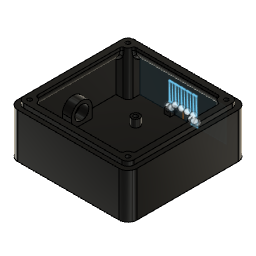
CO2 Melder RG Projekt 2 überarbeitung v13 (Autodesk Fusion 360 design; units mm, degrees)
Autodesk Fusion 360 part; units mm, degrees
sketch "Skizze1" plane through (0, 0, 0) normal (0, 0, 1) x (1, 0, 0)
  line L0 (0, 0) -> (80, 0)
  line L1 (80, 0) -> (80, 80)
  line L2 (80, 80) -> (0, 80)
  line L3 (0, 80) -> (0, 0)
  dimension "d1" = 80
  dimension "d2" = 80
  constraint horizontal L0
  constraint vertical L1
  constraint horizontal L2
  constraint vertical L3
  constraint coincident L0.start L3.end
  measures "d1" distance of L0.start L0.end
  measures "d2" distance of L0.start L2.end
extrude "Extrusion1" add sketch "Skizze1" along normal blind 30
shell "Schale1" thickness 3 removed faces 1 at (26.6667, 53.3333, 30)
sketch "Skizze2" plane through (0, 0, 3) normal (0, 0, 1) x (-1, 0, 0)
  line L0 (-3, -77) -> (-3, -3)
  line L1 (-3, -3) -> (-77, -3)
  line L2 (-77, -3) -> (-77, -77)
  line L3 (-77, -77) -> (-3, -77)
  line L4 (-27.15, -58) -> (-52.85, -58) construction
  line L5 (-52.85, -58) -> (-52.85, -5.7) construction
  line L6 (-52.85, -5.7) -> (-27.15, -5.7) construction
  line L7 (-27.15, -5.7) -> (-27.15, -58) construction
  circle A0 centre (-27.15, -58) radius 1.4
  circle A1 centre (-52.85, -58) radius 1.4
  circle A2 centre (-27.15, -5.7) radius 1.4
  circle A3 centre (-52.85, -5.7) radius 1.4
  circle A4 centre (-27.15, -5.7) radius 2.75
  circle A5 centre (-27.15, -58) radius 2.75
  circle A6 centre (-52.85, -58) radius 2.75
  circle A7 centre (-52.85, -5.7) radius 2.75
  line L8 (-3, -3) -> (-77, -77) construction
  line L9 (-3, -3) -> (-5, -5) construction
  line L10 (-3, -3) -> (-18.5563, -18.5563) construction
  line L11 (-77, -77) -> (-61.4437, -61.4437) construction
  circle A8 centre (-18.5563, -18.5563) radius 5
  circle A9 centre (-61.4437, -61.4437) radius 5
  dimension "d7" = 25.7
  dimension "d8" = 52.3
  dimension "d9" = 2.8
  dimension "d10" = 2.8
  dimension "d11" = 2.8
  dimension "d12" = 2.8
  dimension "d13" = 5.5
  dimension "d14" = 5.5
  dimension "d15" = 5.5
  dimension "d16" = 5.5
  dimension "d88" = 22
  dimension "d90" = 22
  dimension "d91" = 10
  dimension "d92" = 10
  constraint horizontal L4
  constraint vertical L5
  constraint horizontal L6
  constraint vertical L7
  constraint coincident L4.start L7.end
  constraint coincident L4.end L5.start
  constraint coincident L6.end L7.start
  constraint coincident L5.end L6.start
  constraint concentric A2 A4
  constraint concentric A0 A5
  constraint concentric A1 A6
  constraint concentric A3 A7
  constraint coincident L0.end L1.start
  constraint coincident L2.end L3.start
  constraint coincident L8 L9.end
  constraint parallel L8 L10
  constraint coincident L10.end A8.centre
  constraint coincident L11.end A9.centre
  measures "d7" distance of L4.start L4.end
  measures "d8" distance of L4.start L6.end
  measures "d9" diameter of A0
  measures "d10" diameter of A1
  measures "d11" diameter of A2
  measures "d12" diameter of A3
  measures "d13" diameter of A4
  measures "d14" diameter of A5
  measures "d15" diameter of A6
  measures "d16" diameter of A7
  measures "d88" distance of L0.end L10.end
  measures "d90" distance of L2.end L11.end
  measures "d91" diameter of A8
  measures "d92" diameter of A9
extrude "Extrusion2" add sketch "Skizze2" along normal blind 5 contours L1 A4 | L1 A4 | L1 A7 | L1 A7 | A5 | A6
extrude "Extrusion11" add sketch "Skizze2" along normal blind 1 contours A8 | A9
fillet "Abrundung1" radius 6 4 edges at (0, 0, 15) (0, 80, 15) (80, 80, 15) (80, 0, 15)
fillet "Abrundung2" radius 4 4 edges at (77, 3, 16.5) (3, 3, 16.5) (3, 77, 16.5) (77, 77, 16.5)
ref_plane "Arbeitsebene1" through (0, 0, 33) normal (0, 0, 1) x (1, 0, 0)
sketch "Skizze3" plane through (40, 40, 33) normal (0, 0, 1) x (1, 0, 0)
  line L0 (-33, -37) -> (33, -37)
  line L1 (37, -33) -> (37, 33)
  line L2 (33, 37) -> (-33, 37)
  line L3 (-37, 33) -> (-37, -33)
  line L4 (-29, -33) -> (29, -33)
  line L5 (33, -29) -> (33, 29)
  line L6 (29, 33) -> (-29, 33)
  line L7 (-33, 29) -> (-33, -29)
  arc A0 (-29, 33) -> (-33, 29) centre (-29, 29) ccw
  arc A1 (-33, -29) -> (-29, -33) centre (-29, -29) ccw
  arc A2 (29, -33) -> (33, -29) centre (29, -29) ccw
  arc A3 (33, 29) -> (29, 33) centre (29, 29) ccw
  arc A4 (-37, -33) -> (-33, -37) centre (-33, -33) ccw
  arc A5 (33, -37) -> (37, -33) centre (33, -33) ccw
  arc A6 (37, 33) -> (33, 37) centre (33, 33) ccw
  arc A7 (-33, 37) -> (-37, 33) centre (-33, 33) ccw
  circle A8 centre (-33, -33) radius 1.4
  circle A9 centre (33, -33) radius 1.4
  circle A10 centre (-33, 33) radius 1.4
  circle A11 centre (33, 33) radius 1.4
  line L8 (37, 37) -> (29, 37)
  line L9 (29, 37) -> (29, 32)
  line L10 (32.3, 28.7) -> (37, 28.7)
  line L11 (37, 28.7) -> (37, 37)
  arc A12 (29, 32) -> (32.3, 28.7) centre (32.3, 32) ccw
  line L12 (-37, 37) -> (-29, 37)
  line L13 (-29, 37) -> (-29, 32.3)
  line L14 (-32.3, 29) -> (-37, 29)
  line L15 (-37, 29) -> (-37, 37)
  arc A13 (-32.3, 29) -> (-29, 32.3) centre (-32.3, 32.3) ccw
  line L16 (-32.3, -29) -> (-37, -29)
  line L17 (-37, -29) -> (-37, -37)
  line L18 (-37, -37) -> (-29, -37)
  line L19 (-29, -37) -> (-29, -32.3)
  arc A14 (-29, -32.3) -> (-32.3, -29) centre (-32.3, -32.3) ccw
  line L20 (37, -37) -> (29, -37)
  line L21 (29, -37) -> (29, -32.3)
  line L22 (32.3, -29) -> (37, -29)
  line L23 (37, -29) -> (37, -37)
  arc A15 (32.3, -29) -> (29, -32.3) centre (32.3, -32.3) ccw
  line L24 (-34, 40) -> (34, 40)
  line L25 (40, 34) -> (40, -34)
  line L26 (34, -40) -> (-34, -40)
  line L27 (-40, -34) -> (-40, 34)
  arc A16 (-34, 40) -> (-40, 34) centre (-34, 34) ccw
  arc A17 (40, 34) -> (34, 40) centre (34, 34) ccw
  arc A18 (34, -40) -> (40, -34) centre (34, -34) ccw
  arc A19 (-40, -34) -> (-34, -40) centre (-34, -34) ccw
  point P0 (33, -33)
  point P1 (-33, 33)
  point P2 (-33, -33)
  dimension "d22" = 66
  dimension "d23" = 66
  dimension "d26" = 4
  dimension "d29" = 4
  dimension "d36" = 2.8
  dimension "d37" = 2.8
  dimension "d38" = 2.8
  dimension "d39" = 2.8
  dimension "d48" = 3.3
  dimension "d49" = 3.3
  dimension "d50" = 3.3
  dimension "d51" = 3.3
  dimension "d97" = 6
  constraint horizontal L0
  constraint vertical L1
  constraint horizontal L2
  constraint vertical L3
  constraint horizontal L4
  constraint vertical L5
  constraint horizontal L6
  constraint vertical L7
  constraint coincident P1 L6
  constraint coincident P1 L7
  constraint tangent L6 A0
  constraint tangent L7 A0
  constraint coincident L4 P2
  constraint coincident L7 P2
  constraint tangent L4 A1
  constraint tangent L7 A1
  constraint equal A0 A1
  constraint coincident P0 L4
  constraint coincident P0 L5
  constraint tangent L4 A2
  constraint tangent L5 A2
  constraint equal A0 A2
  constraint tangent L5 A3
  constraint tangent L6 A3
  constraint equal A0 A3
  constraint tangent L0 A4
  constraint tangent L3 A4
  constraint tangent L0 A5
  constraint tangent L1 A5
  constraint equal A4 A5
  constraint tangent L1 A6
  constraint tangent L2 A6
  constraint equal A4 A6
  constraint tangent L2 A7
  constraint tangent L3 A7
  constraint equal A4 A7
  constraint coincident P2 A4.centre
  constraint concentric A5 A9
  constraint coincident P1 A7.centre
  constraint concentric A6 A11
  constraint horizontal L8
  constraint vertical L9
  constraint horizontal L10
  constraint vertical L11
  constraint tangent L9 A12
  constraint tangent L10 A12
  constraint horizontal L12
  constraint vertical L13
  constraint horizontal L14
  constraint vertical L15
  constraint tangent L13 A13
  constraint tangent L14 A13
  constraint horizontal L16
  constraint vertical L17
  constraint horizontal L18
  constraint vertical L19
  constraint tangent L16 A14
  constraint tangent L19 A14
  constraint horizontal L20
  constraint vertical L21
  constraint horizontal L22
  constraint vertical L23
  constraint tangent L21 A15
  constraint tangent L22 A15
  constraint horizontal L24
  constraint vertical L25
  constraint horizontal L26
  constraint vertical L27
  constraint tangent L24 A16
  constraint tangent L27 A16
  constraint tangent L24 A17
  constraint tangent L25 A17
  constraint equal A16 A17
  constraint tangent L25 A18
  constraint tangent L26 A18
  constraint equal A16 A18
  constraint tangent L26 A19
  constraint tangent L27 A19
  constraint equal A16 A19
  measures "d22" distance of P0 P2
  measures "d23" distance of P1 A4.centre
  measures "d26" radius of A0
  measures "d29" radius of A4
  measures "d36" diameter of A8
  measures "d37" diameter of A9
  measures "d38" diameter of A10
  measures "d39" diameter of A11
  measures "d48" radius of A12
  measures "d49" radius of A13
  measures "d50" radius of A14
  measures "d51" radius of A15
  measures "d97" radius of A16
extrude "Extrusion3" add sketch "Skizze3" against normal blind 8 contours L0 L3 A1 A4 L16 L17 L18 L19 | L0 L4 L19 L21 | L0 L1 A2 A5 L20 L21 L22 L23 | L3 L7 L14 L16 | L2 L3 A0 A7 L12 L13 L14 L15 | L1 L5 L10 L22 | L1 L2 L5 A3 A6 L8 L9 L10 L11 | L2 L6 L9 L13 | A8 | A9 | A10 | A11
extrude "Extrusion4" add sketch "Skizze3" against normal blind 30 contours L0 L3 A1 A4 L16 L17 L18 L19 | L0 L1 A2 A5 L20 L21 L22 L23 | A1 L16 L19 A14 | A2 L21 L22 A15 | L2 L3 A0 A7 L12 L13 L14 L15 | A0 L13 L14 A13 | L5 A3 L9 L10 A12 | L1 L2 L5 A3 A6 L8 L9 L10 L11
extrude "Extrusion5" cut sketch "Skizze3" against normal blind 10 contours A8 | A9 | A10 | A11
fillet "Abrundung3" radius 6.5 4 edges at (73, 39.85, 25) (40, 73, 25) (40, 7, 25) (7, 40, 25)
fillet "Abrundung4" radius 1.5 16 edges at (11, 73, 32) (11, 74.0917, 27.3944) (7, 69, 32) (5.9083, 69, 27.3944) (73, 11, 32) (74.0917, 11, 27.3944) (69, 7, 32) (69, 5.9083, 27.3944) (11, 7, 32) (11, 5.9083, 27.3944) (7, 11, 32) (5.9083, 11, 27.3944) (69, 73, 32) (69, 74.0917, 27.3944) (73, 68.7, 32) (74.0917, 68.7, 27.3944)
sketch "Skizze4" plane through (3, 0, 0) normal (1, 0, 0) x (0, 1, 0)
  spline S0 degree 3 poles (12.5, 25) (12.319, 25) (12.1066, 24.955) (11.7677, 24.8078) (11.5831, 24.6771) (11.3175, 24.3994) (11.1914, 24.2012) (11.0451, 23.8344) (11, 23.5998) (11, 23.4007) knots 0.456476 0.456476 0.456476 0.456476 0.510767 0.510767 0.567321 0.567321 0.62605 0.62605 0.685782 0.685782 0.685782 0.685782
  line L0 (11, 23.4007) -> (11, 3)
  line L1 (11, 3) -> (69, 3)
  line L2 (69, 3) -> (69, 23.4007)
  spline S1 degree 3 poles (69, 23.4007) (69, 23.5998) (68.9549, 23.8344) (68.8086, 24.2012) (68.6825, 24.3994) (68.4169, 24.6771) (68.2323, 24.8078) (67.8934, 24.955) (67.681, 25) (67.5, 25) knots 0.227171 0.227171 0.227171 0.227171 0.286902 0.286902 0.345632 0.345632 0.402185 0.402185 0.456476 0.456476 0.456476 0.456476
  line L3 (67.5, 25) -> (12.5, 25)
  circle A0 centre (40, 10) radius 7
  circle A1 centre (40, 10) radius 4.75
  circle A2 centre (40, 10) radius 0.9
  line L4 (33, 10) -> (33, 3)
  line L5 (47, 10) -> (47, 3)
  line L6 (33, 3) -> (47, 3)
  dimension "d55" = 9.5
  dimension "d56" = 1.8
  constraint concentric A0 A1
  constraint concentric A0 A2
  constraint coincident L1 L4.end
  constraint coincident L1 L5.end
  constraint perpendicular L5 L6
  measures "d55" diameter of A1
  measures "d56" diameter of A2
extrude "Extrusion6" add sketch "Skizze4" along normal blind 6 contours L1 A0 L4 L6 | L1 A0 L5 L6 | A0
extrude "Extrusion7" cut sketch "Skizze4" against normal blind 3 contours A2
sketch "Skizze5" plane through (0, 77, 0) normal (0, -1, 0) x (1, 0, 0)
  spline S0 degree 3 poles (69, 23.4007) (69, 23.5998) (68.9549, 23.8344) (68.8086, 24.2012) (68.6825, 24.3994) (68.4169, 24.6771) (68.2323, 24.8078) (67.8934, 24.955) (67.681, 25) (67.5, 25) knots 0.227171 0.227171 0.227171 0.227171 0.286902 0.286902 0.345632 0.345632 0.402185 0.402185 0.456476 0.456476 0.456476 0.456476
  line L0 (67.5, 25) -> (12.5, 25)
  spline S1 degree 3 poles (12.5, 25) (12.319, 25) (12.1066, 24.955) (11.7677, 24.8078) (11.5831, 24.6771) (11.3175, 24.3994) (11.1914, 24.2012) (11.0451, 23.8344) (11, 23.5998) (11, 23.4007) knots 0.456476 0.456476 0.456476 0.456476 0.510767 0.510767 0.567321 0.567321 0.62605 0.62605 0.685782 0.685782 0.685782 0.685782
  line L1 (11, 23.4007) -> (11, 3)
  line L2 (11, 3) -> (69, 3)
  line L3 (69, 3) -> (69, 23.4007)
  line L4 (31, 21) -> (49, 21)
  line L5 (49, 21) -> (49, 9)
  line L6 (49, 9) -> (31, 9)
  line L7 (31, 9) -> (31, 21)
  line L8 (31, 21) -> (33, 21)
  line L9 (33, 21) -> (33, 9)
  line L10 (33, 9) -> (31, 9)
  line L11 (31, 9) -> (31, 21)
  line L12 (37, 9) -> (35, 9)
  line L13 (35, 9) -> (35, 21)
  line L14 (35, 9) -> (35, 21)
  line L15 (37, 21) -> (37, 9)
  line L16 (35, 21) -> (37, 21)
  line L17 (41, 9) -> (39, 9)
  line L18 (39, 9) -> (39, 21)
  line L19 (39, 9) -> (39, 21)
  line L20 (41, 21) -> (41, 9)
  line L21 (39, 21) -> (41, 21)
  line L22 (45, 9) -> (43, 9)
  line L23 (43, 9) -> (43, 21)
  line L24 (43, 9) -> (43, 21)
  line L25 (45, 21) -> (45, 9)
  line L26 (43, 21) -> (45, 21)
  line L27 (49, 9) -> (47, 9)
  line L28 (47, 9) -> (47, 21)
  line L29 (47, 9) -> (47, 21)
  line L30 (49, 21) -> (49, 9)
  line L31 (47, 21) -> (49, 21)
  line L32 (40, 3) -> (34.4, 3) construction
  line L33 (40, 3) -> (40, 3.3884) construction
  line L34 (40, 3.3884) -> (40, 9) construction
  line L35 (34.4, 3) -> (30.4, 3)
  line L36 (30.4, 3) -> (30.4, 6)
  line L37 (34.4, 6) -> (34.4, 3)
  circle A0 centre (32.4, 6) radius 0.95
  circle A1 centre (32.4, 6) radius 2
  circle A2 centre (47.6, 6) radius 0.95
  line L38 (49.6, 3) -> (49.6, 6)
  circle A3 centre (47.6, 6) radius 2
  line L39 (45.6, 6) -> (45.6, 3)
  line L40 (45.6, 3) -> (49.6, 3)
  dimension "d64" = 18
  dimension "d65" = 12
  dimension "d68" = 16
  dimension "d69" = 0
  dimension "d70" = 5.6
  dimension "d71" = 4
  dimension "d72" = 3
  dimension "d73" = 1.9
  dimension "d74" = 4
  constraint horizontal L4
  constraint vertical L5
  constraint horizontal L6
  constraint vertical L7
  constraint horizontal L8
  constraint vertical L9
  constraint horizontal L10
  constraint vertical L11
  constraint midpoint L2 L32.start
  constraint parallel L2 L32
  constraint perpendicular L2 L33
  constraint midpoint L6 L34.end
  constraint horizontal L35
  constraint vertical L36
  constraint vertical L37
  constraint concentric A0 A1
  constraint symmetric L32.end L34 L39.end
  constraint symmetric L34 L35.end L38.start
  constraint symmetric L34 L36.end L38.end
  constraint symmetric L34 L37.start L39.start
  constraint symmetric L34 A0 A2
  constraint symmetric L34 A1 A3
  measures "d64" distance of L4.start L4.end
  measures "d65" distance of L4.start L6.end
  measures "d70" distance of L32.start L32.end
  measures "d71" distance of L32.end L35.end
  measures "d72" distance of L32.end L37.start
  measures "d73" diameter of A0
  measures "d74" diameter of A1
extrude "Extrusion8" add sketch "Skizze5" along normal blind 3 contours L2 L38 A3 L39 L40 | A3 | L2 L35 L36 L37 A1 | A1
extrude "Extrusion9" [suppressed]
fillet "Abrundung5" [suppressed]
sketch "Skizze6" plane through (0, 0, 0) normal (0, -1, 0) x (1, 0, 0)
  line L0 (74, 0) -> (74, 30)
  line L1 (74, 30) -> (6, 30)
  line L2 (6, 30) -> (6, 0)
  line L3 (6, 0) -> (74, 0)
  line L4 (36.5, 8.5154) -> (43.5, 8.5154)
  line L5 (44.5, 9.5154) -> (44.5, 12.0154)
  line L6 (43.5, 13.0154) -> (36.5, 13.0154)
  line L7 (35.5, 12.0154) -> (35.5, 9.5154)
  arc A0 (35.5, 9.5154) -> (36.5, 8.5154) centre (36.5, 9.5154) ccw
  arc A1 (36.5, 13.0154) -> (35.5, 12.0154) centre (36.5, 12.0154) ccw
  arc A2 (44.5, 12.0154) -> (43.5, 13.0154) centre (43.5, 12.0154) ccw
  arc A3 (43.5, 8.5154) -> (44.5, 9.5154) centre (43.5, 9.5154) ccw
  point P0 (35.5, 8.5154)
  point P1 (44.5, 8.5154)
  point P2 (35.5, 13.0154)
  point P3 (40, 8.5154)
  point P4 (40, 8.5154)
  dimension "d83" = 9
  dimension "d84" = 4.5
  dimension "d85" = 1
  constraint horizontal L4
  constraint vertical L5
  constraint horizontal L6
  constraint vertical L7
  constraint coincident P0 L4
  constraint coincident P0 L7
  constraint tangent L4 A0
  constraint tangent L7 A0
  constraint coincident P2 L6
  constraint coincident P2 L7
  constraint tangent L6 A1
  constraint tangent L7 A1
  constraint equal A0 A1
  constraint tangent L5 A2
  constraint tangent L6 A2
  constraint equal A0 A2
  constraint coincident P1 L4
  constraint coincident P1 L5
  constraint tangent L4 A3
  constraint tangent L5 A3
  constraint equal A0 A3
  constraint midpoint L4 P4
  measures "d83" distance of P0 P1
  measures "d84" distance of P0 P2
  measures "d85" radius of A0
extrude "Extrusion10" [suppressed]
sketch "Skizze7" plane through (0, 0, 0) normal (0, 0, -1) x (1, 0, 0)
  arc A0 (80, -6) -> (74, 0) centre (74, -6) ccw
  line L0 (74, 0) -> (6, 0)
  arc A1 (6, 0) -> (0, -6) centre (6, -6) ccw
  line L1 (0, -6) -> (0, -74)
  arc A2 (0, -74) -> (6, -80) centre (6, -74) ccw
  line L2 (6, -80) -> (74, -80)
  arc A3 (74, -80) -> (80, -74) centre (74, -74) ccw
  line L3 (80, -74) -> (80, -6)
  spline S0 degree 3 poles (40.0131, -5.2) (59.3523, -5.2) (74.7984, -20.6974) (74.7053, -40.2042) knots 0 0 0 0 1 1 1 1
  spline S1 degree 3 poles (74.7053, -40.2042) (74.6005, -59.3757) (59.0798, -74.1629) (40.8653, -74.603) knots 0 0 0 0 1 1 1 1
  spline S2 degree 3 poles (40.8653, -74.603) (21.7986, -75.0686) (5.2767, -59.8995) (5.3, -39.8596) knots 0 0 0 0 1 1 1 1
  spline S3 degree 3 poles (5.3, -39.8596) (5.3233, -19.8196) (21.7241, -5.0254) (40.0131, -5.2) knots 0 0 0 0 1 1 1 1
  spline S4 degree 3 poles (40.0178, -72.1093) (22.8393, -72.2118) (7.7564, -58.3116) (7.7843, -39.8456) knots 0 0 0 0 1 1 1 1
  spline S5 degree 3 poles (7.7843, -39.8456) (7.8123, -21.2841) (23.0582, -7.5423) (40.1901, -7.6541) knots 0 0 0 0 1 1 1 1
  spline S6 degree 3 poles (40.1901, -7.6541) (57.7154, -7.7612) (72.2559, -22.1968) (72.2419, -39.6593) knots 0 0 0 0 1 1 1 1
  spline S7 degree 3 poles (72.2419, -39.6593) (72.2279, -57.6783) (57.8994, -72.1093) (40.0178, -72.1093) knots 0 0 0 0 1 1 1 1
  spline S8 degree 3 poles (65.6248, -39.8922) (65.662, -53.9576) (54.1694, -65.5341) (40.1249, -65.5294) knots 0 0 0 0 1 1 1 1
  arc A4 (40.1249, -65.5294) -> (14.3805, -40.5441) centre (39.9845, -39.9182) cw
  spline S9 degree 3 poles (14.3805, -40.5441) (14.0382, -26.2831) (25.3237, -14.3899) (39.7151, -14.2805) knots 0 0 0 0 1 1 1 1
  arc A5 (39.7151, -14.2805) -> (65.6248, -39.8922) centre (40.0761, -39.8268) cw
  line L4 (60.6072, -50.4744) -> (47.3776, -42.6862)
  arc A6 (47.3776, -37.1471) -> (47.3776, -42.6862) centre (39.6022, -39.9166) cw
  line L5 (47.3776, -37.1471) -> (60.6491, -29.3891)
  spline S10 degree 3 poles (60.6491, -29.3891) (63.974, -36.4369) (63.974, -43.408) (60.6072, -50.4744) knots 0 0 0 0 1 1 1 1
  line L6 (38.6813, -16.8673) -> (38.6813, -32.1155)
  arc A7 (33.9385, -34.8932) -> (38.6813, -32.1155) centre (40.1695, -40.0945) cw
  line L7 (33.9385, -34.8932) -> (20.7229, -27.2516)
  spline S11 degree 3 poles (20.7229, -27.2516) (24.3597, -21.1142) (32.1038, -16.9045) (38.6813, -16.8673) knots 0 0 0 0 1 1 1 1
  line L8 (19.3957, -29.5125) -> (32.5974, -37.1517)
  spline S12 degree 3 poles (32.5974, -37.1517) (32.0386, -38.9888) (31.978, -40.8049) (32.637, -42.6582) knots 0 0 0 0 1 1 1 1
  line L9 (32.637, -42.6582) -> (19.4376, -50.3417)
  spline S13 degree 3 poles (19.4376, -50.3417) (16.0546, -44.316) (16.0103, -35.7012) (19.3957, -29.5125) knots 0 0 0 0 1 1 1 1
  arc A8 (38.672, -47.6455) -> (33.9967, -44.9935) centre (40.1301, -39.6279) cw
  line L10 (38.672, -47.6455) -> (38.672, -62.8845)
  spline S14 degree 3 poles (38.672, -62.8845) (33.2423, -63.583) (23.2142, -57.811) (20.7648, -52.5886) knots 0 0 0 0 1 1 1 1
  line L11 (20.7648, -52.5886) -> (33.878, -44.9935)
  spline S15 degree 3 poles (33.878, -44.9935) (33.8966, -44.9819) (33.9385, -44.9935) (33.9967, -44.9935) knots 0 0 0 0 1 1 1 1
  spline S16 degree 3 poles (41.3705, -16.7695) (48.9795, -17.4098) (54.8749, -20.8534) (59.3243, -27.1166) knots 0 0 0 0 1 1 1 1
  line L12 (59.3243, -27.1166) -> (46.0738, -34.8606)
  arc A9 (41.3705, -32.1458) -> (46.0738, -34.8606) centre (39.8921, -40.1384) cw
  line L13 (41.3705, -32.1458) -> (41.3705, -16.7695)
  spline S17 degree 3 poles (41.3892, -47.6898) (43.8712, -46.9167) (44.1692, -46.7421) (46.0924, -44.954) knots 0 0 0 0 1 1 1 1
  line L14 (46.0924, -44.954) -> (59.2847, -52.7329)
  spline S18 degree 3 poles (59.2847, -52.7329) (54.8795, -58.9379) (48.9865, -62.3722) (41.3892, -63.0125) knots 0 0 0 0 1 1 1 1
  line L15 (41.3892, -63.0125) -> (41.3892, -47.6898)
  arc A10 (34.637, -39.8503) -> (40.1086, -34.5207) centre (40.0428, -39.9267) cw
  spline S19 degree 3 poles (40.1086, -34.5207) (42.9608, -34.5486) (45.3846, -37.012) (45.3916, -39.8898) knots 0 0 0 0 1 1 1 1
  arc A11 (45.3916, -39.8898) -> (34.637, -39.8503) centre (40.0139, -39.9802) cw
  point P0 (40, -40)
extrude "Extrusion12" [suppressed]
extrude "Extrusion13" [suppressed]
equation "d70 = 5.85 mm - 0.25 mm"
named bodies: "Gehaeuse 80x80", "Plexi Glas 80x80"
